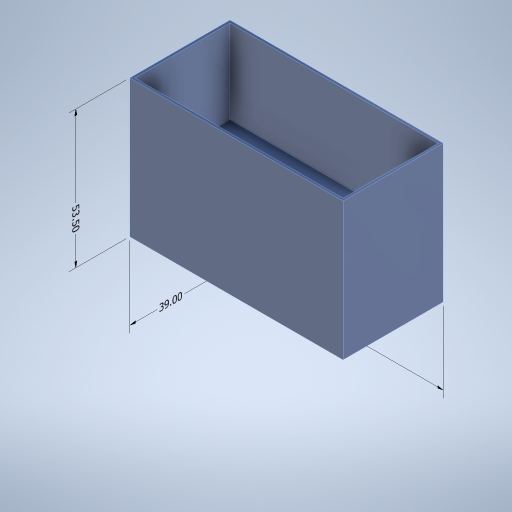
# Autodesk Inventor part: Capsula
Saved by Autodesk Inventor 2023 (Build 270158000, 158)
## iProperties
Created: 2023-03-19
Part Number: Capsula
Material: Plástico PET
Document SubType Name: Modeling
Designer: sergi
Density: 1.541 g/cm^3
Appearance: Satinado con motas - Azul
Author: sergi
Autodesk Inventor part; units mm, degrees
ref_plane "YZ Plane" through (0, 0, 0) normal (1, 0, 0) x (0, 1, 0)
ref_plane "XZ Plane" through (0, 0, 0) normal (0, 1, 0) x (-1, 0, 0)
ref_plane "XY Plane" through (0, 0, 0) normal (0, 0, 1) x (1, 0, 0)
sketch "Boceto1" plane through (0, 0, 0) normal (0, 1, 0) x (-1, 0, 0)
  line L0 (-41.5, 19.5) -> (41.5, 19.5)
  line L1 (41.5, 19.5) -> (41.5, -19.5)
  line L2 (41.5, -19.5) -> (-41.5, -19.5)
  line L3 (-41.5, -19.5) -> (-41.5, 19.5)
  line L4 (-41.5, 19.5) -> (41.5, -19.5) construction
  line L5 (41.5, 19.5) -> (-41.5, -19.5) construction
  line L6 (-40.5, 18.5) -> (40.5, 18.5)
  line L7 (40.5, 18.5) -> (40.5, -18.5)
  line L8 (40.5, -18.5) -> (-40.5, -18.5)
  line L9 (-40.5, -18.5) -> (-40.5, 18.5)
  line L10 (-40.5, 18.5) -> (40.5, -18.5) construction
  line L11 (40.5, 18.5) -> (-40.5, -18.5) construction
  point P0 (0, 0)
  dimension "d0" = 83
  dimension "d1" = 39
  dimension "d2" = 1
  dimension "d3" = 1
  constraints: 24 end point, 4 midpoint, 4 parallel, 2 horizontal, 2 perpendicular
  measures "d0" distance of L1.end L2.end
  measures "d1" distance of L0.end L1.end
  measures "d2" distance between parallel lines of L1 L7
  measures "d3" distance between parallel lines of L2 L8
extrude "Extrusión1" add sketch "Boceto1" along normal blind 3 contours L6 L7 L8 L9
extrude "Extrusión2" add sketch "Boceto1" along normal blind 20
sketch "Boceto2" plane through (0, 20, 0) normal (0, 1, 0) x (1, 0, 0)
  line L0 (41.5, 19.5) -> (-41.5, 19.5) projected
  line L1 (41.5, -19.5) -> (-41.5, -19.5)
  line L2 (-41.5, -19.5) -> (-41.5, 19.5)
  line L3 (-41.5, 19.5) -> (41.5, 19.5)
  line L4 (41.5, 19.5) -> (41.5, -19.5)
  line L5 (41.5, -19.5) -> (-41.5, 19.5) construction
  line L6 (-41.5, -19.5) -> (41.5, 19.5) construction
  line L7 (35.5, -13.5) -> (-35.5, -13.5)
  line L8 (-35.5, -13.5) -> (-35.5, 13.5)
  line L9 (-35.5, 13.5) -> (35.5, 13.5)
  line L10 (35.5, 13.5) -> (35.5, -13.5)
  line L11 (35.5, -13.5) -> (-35.5, 13.5) construction
  line L12 (-35.5, -13.5) -> (35.5, 13.5) construction
  point P0 (0, 0)
  dimension "d8" = 6
  dimension "d9" = 6
  constraints: 24 end point, 4 midpoint, 4 parallel, 2 horizontal, 2 perpendicular
  measures "d8" distance between parallel lines of L2 L8
  measures "d9" distance between parallel lines of L0 L9
extrude "Extrusión3" add sketch "Boceto2" along normal blind 1
sketch "Boceto3" plane through (0, 21, 0) normal (0, 1, 0) x (1, 0, 0)
  point P0 (0, 0)
sketch "Boceto4" plane through (0, 21, 0) normal (0, 1, 0) x (1, 0, 0)
  line L0 (-41.5, 19.5) -> (-41.5, -19.5) projected
  line L1 (41.5, -19.5) -> (-41.5, -19.5)
  line L2 (-41.5, -19.5) -> (-41.5, 19.5)
  line L3 (-41.5, 19.5) -> (41.5, 19.5)
  line L4 (41.5, 19.5) -> (41.5, -19.5)
  line L5 (41.5, -19.5) -> (-41.5, 19.5) construction
  line L6 (-41.5, -19.5) -> (41.5, 19.5) construction
  line L7 (40.5, -18.5) -> (-40.5, -18.5)
  line L8 (-40.5, -18.5) -> (-40.5, 18.5)
  line L9 (-40.5, 18.5) -> (40.5, 18.5)
  line L10 (40.5, 18.5) -> (40.5, -18.5)
  line L11 (40.5, -18.5) -> (-40.5, 18.5) construction
  line L12 (-40.5, -18.5) -> (40.5, 18.5) construction
  point P0 (0, 0)
  point P1 (-41.5, -19.5)
  dimension "d21" = 1
  dimension "d22" = 1
  constraints: 24 end point, 4 midpoint, 4 parallel, 2 horizontal, 2 perpendicular
  measures "d21" distance between parallel lines of L0 L8
  measures "d22" distance between parallel lines of L3 L9
extrude "Extrusión4" add sketch "Boceto4" along normal blind 32.5
